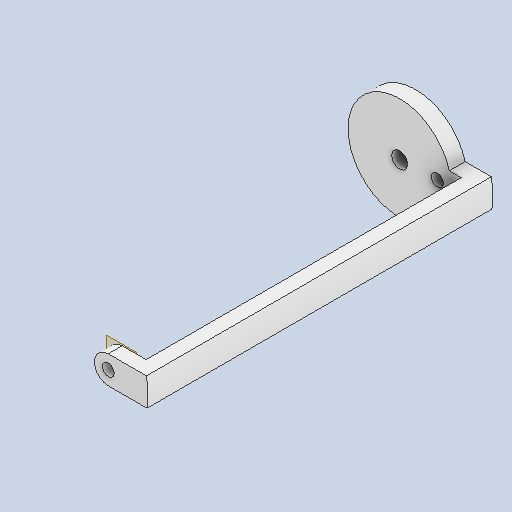
# Autodesk Inventor part: Part11
Saved by Autodesk Inventor 2022.3 (Build 263350000, 350)
## iProperties
Created: 2022-11-16
Part Number: Part11
Material: PC/ABS Plastic
Document SubType Name: Modeling
Designer: komputer
Density: 0.357273 g/cm^3
Appearance: Smooth - White
Mass: 1.59898 g
Surface Area: 35.4884 cm^2
Volume: 4.47553 cm^3
Author: komputer
Autodesk Inventor part; units mm, degrees
ref_plane "YZ Plane" through (0, 0, 0) normal (1, 0, 0) x (0, 1, 0)
ref_plane "XZ Plane" through (0, 0, 0) normal (0, 1, 0) x (-1, 0, 0)
ref_plane "Work Plane1" through (-0.1632, 0, 0) normal (0, 0, 1) x (1, 0, 0)
sketch "Sketch1" plane through (-0.1632, 0, 0) normal (0, 0, 1) x (1, 0, 0)
  circle A0 centre (9.6632, 0) radius 1.5 projected
  line L0 (12.6832, 3.5) -> (9.6632, 3.5) projected
  arc A1 (9.6632, 3.5) -> (9.6632, -3.5) centre (9.6632, 0) ccw projected
  line L1 (9.6632, -3.5) -> (12.6832, -3.5) projected
  arc A2 (12.6832, -3.5) -> (12.6832, 3.5) centre (0.1632, 0) ccw projected
  circle A3 centre (0.1788, -0.3768) radius 14 projected
  circle A4 centre (0.1788, -0.3768) radius 11 projected
  line L2 (12.6832, -3.5) -> (18.2293, -3.5)
  line L3 (12.6832, 3.5) -> (18.7282, 3.5)
  circle A5 centre (0.1788, -0.3768) radius 16.5
  line L4 (16.6788, -0.3768) -> (20.6788, -0.3768)
  circle A6 centre (0.1788, -0.3768) radius 20.5
  line L5 (18.7282, 3.5) -> (20.3088, 3.5)
  line L6 (18.2293, -3.5) -> (20.4394, -3.5)
  point P0 (0.1632, 0)
  dimension "d0" = 33
  dimension "d1" = 4
  constraints: 10 end point, 5 horizontal, 3 point on circle, 2 coincident, 2 collinear, 1 centre point, 1 horizontal alignment, 1 parallel, 2 other
  measures "d1" distance of L4.start L4.end
extrude "Extrusion1" add sketch "Sketch1" along normal blind 3.5 contours A2 L1 A4 L0 | L3 A3 L2 A2 | A4 L1 A1 L0 | L3 A5 L2 A3 | L3 L5 A6 L4 A5 | A5 L4 A6 L6 L2 picked at (10.1281, -2.4909) picked at (14.5943, 3.0756)
sketch "Sketch2" plane through (-0.1632, 0, 0) normal (0, 0, -1) x (-1, 0, 0)
  line L0 (-9.6632, -3.5) -> (-20.4394, -3.5) projected
  arc A0 (-9.6632, -3.5) -> (-9.6632, 3.5) centre (-9.6632, 0) ccw projected
  line L1 (-20.3088, 3.5) -> (-9.6632, 3.5) projected
  arc A1 (-20.3088, 3.5) -> (-20.4394, -3.5) centre (-0.1788, -0.3768) ccw projected
  circle A2 centre (-9.6632, 0) radius 1.5 projected
  circle A3 centre (-0.1788, -0.3768) radius 14 projected
  line L2 (-14.1788, -0.3768) -> (-16.1788, -0.3768)
  circle A4 centre (-0.1788, -0.3768) radius 16
  line L3 (-16.1788, -0.3768) -> (-19.6788, -0.3768)
  circle A5 centre (-0.1788, -0.3768) radius 19.5
  circle A6 centre (-0.1788, -0.3768) radius 2 projected
  point P0 (-0.1632, 0)
  point P1 (-19.427, -3.5)
  point P2 (-15.871, -3.5)
  point P3 (-15.702, 3.5)
  point P4 (-19.2895, 3.5)
  dimension "d4" = 2
  dimension "d5" = 3.5
  constraints: 4 end point, 2 coincident, 2 horizontal, 1 horizontal alignment, 7 other
  measures "d4" distance of L2.start L2.end
  measures "d5" distance of L2.end L3.end
ref_plane "Work Plane2" through (-13.9845, -14.3768, -78) normal (0, 0, -1) x (0, 1, 0)
extrude "Extrusion2" add sketch "Sketch2" along normal blind 83.5 contours L0 A5 L3 A4 | L3 A5 L1 A4
sketch "Sketch3" plane through (-0.1632, 0, -83.5) normal (0, 0, -1) x (-1, 0, 0)
  circle A0 centre (-0.1788, -0.3768) radius 14 projected
  circle A1 centre (-9.6632, 0) radius 1.5 projected
  arc A2 (-15.702, 3.5) -> (-15.871, -3.5) centre (-0.1788, -0.3768) ccw projected
  line L0 (-9.6632, -3.5) -> (-15.871, -3.5) projected
  arc A3 (-9.6632, -3.5) -> (-9.6632, 3.5) centre (-9.6632, 0) ccw projected
  line L1 (-15.702, 3.5) -> (-9.6632, 3.5) projected
  circle A4 centre (-0.1788, -0.3768) radius 2
  arc A5 (-9.6632, -3.5) -> (-9.6632, 3.5) centre (-9.6632, 0) ccw projected
  line L2 (-9.6632, 3.5) -> (-12.6832, 3.5) projected
  arc A6 (-12.6832, -3.5) -> (-12.6832, 3.5) centre (-0.1632, 0) ccw projected
  line L3 (-12.6832, -3.5) -> (-9.6632, -3.5) projected
  line L4 (3.8368, -5) -> (-4.1632, -5) projected
  line L5 (3.8368, 5) -> (3.8368, -5) projected
  line L6 (-4.1632, 5) -> (3.8368, 5) projected
  line L7 (-4.1632, -5) -> (-4.1632, 5) projected
  point P0 (-0.1632, 0)
  dimension "d8" = 4
  constraints: 1 centre point, 1 coincident
  measures "d8" diameter of A4
extrude "Extrusion3" add sketch "Sketch3" against normal blind 4 contours L1 A3 L0 A0 | A0 L0 A2 L1 | A6 L0 A3 L1 | L4 L7 L6 L5
sketch "Sketch4" plane through (-0.1632, 0, 3.5) normal (0, 0, 1) x (1, 0, 0)
  arc A0 (19.427, -3.5) -> (19.2895, 3.5) centre (0.1788, -0.3768) ccw projected
  arc A1 (19.427, -3.5) -> (19.2895, 3.5) centre (0.1788, -0.3768) ccw projected
  arc A2 (15.871, -3.5) -> (15.702, 3.5) centre (0.1788, -0.3768) ccw projected
  line L0 (9.6632, -3.5) -> (20.4394, -3.5) projected
  arc A3 (20.4394, -3.5) -> (20.3088, 3.5) centre (0.1788, -0.3768) ccw projected
  line L1 (20.3088, 3.5) -> (9.6632, 3.5) projected
  arc A4 (9.6632, 3.5) -> (9.6632, -3.5) centre (9.6632, 0) ccw projected
  circle A5 centre (9.6632, 0) radius 1.5 projected
  point P0 (0.1632, 0)
  point P1 (19.2895, 3.5)
  point P2 (19.427, -3.5)
extrude "Extrusion4" cut sketch "Sketch4" against normal blind 4 contours A0 L1 A3 L0
body "Solid1"
